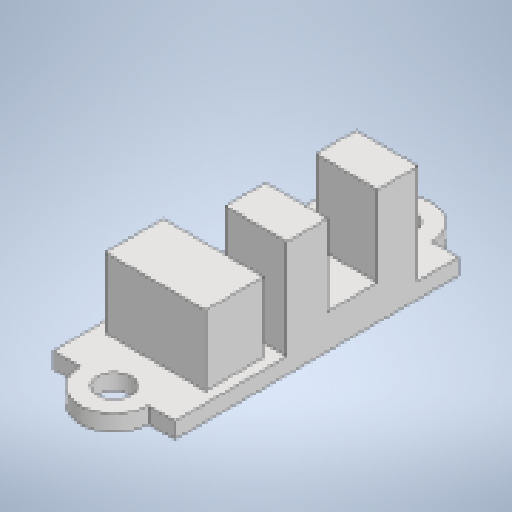
# Autodesk Inventor part: optic endstop module
Saved by Autodesk Inventor 2025 (Build 290162000, 162)
## iProperties
Created: 2025-07-09
Part Number: optic endstop module
Material: 一般
Document SubType Name: Modeling
Designer: gavin
Density: 1 g/cm^3
Appearance: 預設
Author: gavin
Autodesk Inventor part; units mm, degrees
ref_plane "YZ Plane" through (0, 0, 0) normal (1, 0, 0) x (0, 1, 0)
ref_plane "XZ Plane" through (0, 0, 0) normal (0, 1, 0) x (-1, 0, 0)
ref_plane "XY Plane" through (0, 0, 0) normal (0, 0, 1) x (1, 0, 0)
sketch "草圖1" plane through (0, 0, 0) normal (0, 1, 0) x (-1, 0, 0)
  line L0 (6, 14) -> (6, -14)
  line L1 (-6, -14) -> (-6, 14)
  line L2 (-6, 14) -> (6, -14) construction
  line L3 (6, 14) -> (-6, -14) construction
  circle A0 centre (0, 14) radius 1.65
  circle A1 centre (0, -14) radius 1.65
  arc A2 (-3.35, -14) -> (3.35, -14) centre (0, -14) ccw
  arc A3 (3.35, 14) -> (-3.35, 14) centre (0, 14) ccw
  line L4 (-6, 14) -> (-3.35, 14)
  line L5 (1.65, 14) -> (6, 14)
  line L6 (6, -14) -> (3.35, -14)
  line L7 (-3.35, -14) -> (-6, -14)
  point P0 (0, 0)
  dimension "d2" = 3.3
  dimension "d0" = 12
  dimension "d1" = 28
  dimension "d3" = 3.3
  dimension "d4" = 6.7
  dimension "d5" = 6.7
  constraints: 16 end point, 5 parallel, 4 point on circle, 3 centre point, 2 coincident, 2 horizontal, 2 midpoint, 2 perpendicular, 1 horizontal alignment, 1 point on line, 2 other
  measures "d0" distance of L0.end L1.start
  measures "d1" distance of L0.start L0.end
  measures "d3" diameter of A1
  measures "d4" diameter of A2
  measures "d5" diameter of A3
extrude "擠出1" add sketch "草圖1" along normal blind 1.58
sketch "草圖2" plane through (6, 0, 14) normal (1, 0, 0) x (0, 0, -1)
  line L0 (0, 0) -> (28, 0) projected
  line L1 (28, 0) -> (28, 1.58) projected
  line L2 (0, 1.58) -> (28, 1.58) projected
  line L3 (0, 0) -> (0, 1.58) projected
  line L4 (11.06, 1.58) -> (11.06, 11.38)
  line L5 (11.06, 11.38) -> (15.06, 11.38)
  line L6 (15.06, 11.38) -> (15.06, 3.42)
  line L7 (15.06, 3.42) -> (20, 3.42)
  line L8 (20, 3.42) -> (20, 11.38)
  line L9 (20, 11.38) -> (24, 11.38)
  line L10 (24, 11.38) -> (24, 1.58)
  point P0 (14, 0)
  dimension "d8" = 12.94
  dimension "d9" = 4
  dimension "d10" = 4
  dimension "d11" = 4
  dimension "d12" = 7.96
  dimension "d13" = 9.8
  constraints: 14 end point, 5 perpendicular, 4 point on line, 1 vertical
  measures "d8" distance between parallel lines of L10 L4
  measures "d9" distance between parallel lines of L1 L10
  measures "d10" distance of L8.end L9.end
  measures "d11" distance of L4.end L5.end
  measures "d12" distance of L7.end L8.end
  measures "d13" distance of L9.end L10.end
extrude "擠出2" add sketch "草圖2" against normal blind 6.1 contours L4 L5 L6 L7 L8 L9 L10 L2
sketch "草圖3" plane through (0, 1.58, 0) normal (0, 1, 0) x (1, 0, 0)
  line L0 (4.95, -9.93) -> (-4.95, -9.93)
  line L1 (-4.95, -9.93) -> (-4.95, -4.21)
  line L2 (-4.95, -4.21) -> (4.95, -4.21)
  line L3 (4.95, -4.21) -> (4.95, -9.93)
  line L4 (4.95, -9.93) -> (-4.95, -4.21) construction
  line L5 (-4.95, -9.93) -> (4.95, -4.21) construction
  line L6 (6, -2.94) -> (-0.1, -2.94) projected
  line L7 (0, 0) -> (0, -12.3322) construction
  point P0 (0, -7.07)
  dimension "d16" = 1.27
  dimension "d17" = 5.72
  dimension "d18" = 9.9
  constraints: 14 end point, 2 midpoint, 2 parallel, 1 horizontal, 1 perpendicular, 1 point on line, 1 vertical
  measures "d16" distance between parallel lines of L6 L2
  measures "d17" distance of L0.end L1.end
  measures "d18" distance of L0.start L0.end
extrude "擠出3" add sketch "草圖3" along normal blind 6.92
